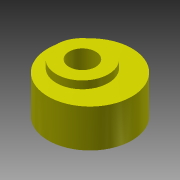
# Autodesk Inventor part: eccentric stop
Saved by Autodesk Inventor 2013 (Build 170138000, 138)
## iProperties
Created: 2013-09-11
Part Number: eccentric stop
Material: Generic
Document SubType Name: Modeling
Designer: employee
Density: 1 g/cm^3
Author: employee
Autodesk Inventor part; units mm, degrees
ref_plane "YZ Plane" through (0, 0, 0) normal (1, 0, 0) x (0, 1, 0)
ref_plane "XZ Plane" through (0, 0, 0) normal (0, 1, 0) x (-1, 0, 0)
ref_plane "XY Plane" through (0, 0, 0) normal (0, 0, 1) x (1, 0, 0)
sketch "Sketch1" plane through (0, 0, 0) normal (0, 0, 1) x (1, 0, 0)
  circle A0 centre (0, 0) radius 5.5
  dimension "d0" = 11
  constraints: 1 centre point, 1 coincident
  measures "d0" diameter of A0
extrude "Extrusion1" add sketch "Sketch1" along normal blind 5
sketch "Sketch2" plane through (0, 0, 5) normal (0, 0, 1) x (1, 0, 0)
  circle A0 centre (0, 0) radius 5.5 projected
  line L0 (0, 0) -> (-1, 0)
  circle A1 centre (-1, 0) radius 1.75
  circle A2 centre (-1, 0) radius 3.4167
  dimension "d5" = 1
  dimension "d6" = 3.5
  dimension "d7" = 1.6667
  constraints: 2 centre point, 2 coincident, 2 end point, 1 horizontal
  measures "d5" distance of L0.start L0.end
  measures "d6" diameter of A1
  measures "d7" radial gap between concentric circles of A1 A2
extrude "Extrusion2" add sketch "Sketch2" along normal blind 1 contours A2
sketch "Sketch3" plane through (-1, 0, 5) normal (0, 0, 1) x (1, 0, 0)
  circle A0 centre (0, 0) radius 1.75 projected
  point P0 (1, 0)
extrude "Extrusion3" cut sketch "Sketch3" against normal through all
body "Solid1"
